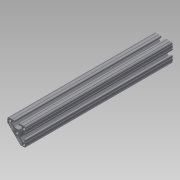
# Autodesk Inventor part: 1547
Saved by Autodesk Inventor 2013 (Build 170138000, 138)
## iProperties
Company: 80/20 Inc.
Created: 2014-04-23
Part Number: 1547
Material: Generic
Document SubType Name: Modeling
Density: 1 g/cm^3
Vendor: 80/20 Inc.
Engineer: Ross Bowman
Designer: Ross Bowman
Catalog Web Link: 8020.net
Material: 6105-T5 Aluminum
Author: Ross Bowman
Keywords: 80/20 , 8020 , T-Slot , Extrusion
Autodesk Inventor part; units mm, degrees
ref_plane "YZ Plane" through (0, 0, 0) normal (1, 0, 0) x (0, 1, 0)
ref_plane "XZ Plane" through (0, 0, 0) normal (0, 1, 0) x (-1, 0, 0)
ref_plane "XY Plane" through (0, 0, 0) normal (0, 0, 1) x (1, 0, 0)
sketch "Sketch1" plane through (0, 0, 0) normal (0, 0, 1) x (1, 0, 0)
  circle A0 centre (0, 0) radius 3.3274
  arc A1 (12.2428, 17.272) -> (11.8618, 16.891) centre (12.2428, 16.891) ccw
  line L0 (14.478, 17.272) -> (12.2428, 17.272)
  arc A2 (17.272, 14.478) -> (14.478, 17.272) centre (14.478, 14.478) ccw
  line L1 (17.272, 12.2682) -> (17.272, 14.478)
  arc A3 (16.891, 11.8872) -> (17.272, 12.2682) centre (16.891, 12.2682) ccw
  line L2 (12.2428, 11.8872) -> (16.891, 11.8872)
  arc A4 (11.8618, 12.2682) -> (12.2428, 11.8872) centre (12.2428, 12.2682) ccw
  line L3 (11.8618, 16.891) -> (11.8618, 12.2682)
  arc A5 (-12.2428, 11.8872) -> (-11.8618, 12.2682) centre (-12.2428, 12.2682) ccw
  line L4 (-16.8656, 11.8872) -> (-12.2428, 11.8872)
  arc A6 (-17.2466, 12.2682) -> (-16.8656, 11.8872) centre (-16.8656, 12.2682) ccw
  line L5 (-17.2466, 14.478) -> (-17.2466, 12.2682)
  arc A7 (-14.4526, 17.272) -> (-17.2466, 14.478) centre (-14.4526, 14.478) ccw
  line L6 (-12.2428, 17.272) -> (-14.4526, 17.272)
  arc A8 (-11.8618, 16.891) -> (-12.2428, 17.272) centre (-12.2428, 16.891) ccw
  line L7 (-11.8618, 12.2682) -> (-11.8618, 16.891)
  arc A9 (14.478, -17.272) -> (17.272, -14.478) centre (14.478, -14.478) ccw
  line L8 (12.2428, -17.272) -> (14.478, -17.272)
  arc A10 (11.8618, -16.891) -> (12.2428, -17.272) centre (12.2428, -16.891) ccw
  line L9 (11.8618, -12.2682) -> (11.8618, -16.891)
  arc A11 (12.2428, -11.8872) -> (11.8618, -12.2682) centre (12.2428, -12.2682) ccw
  line L10 (16.891, -11.8872) -> (12.2428, -11.8872)
  arc A12 (17.272, -12.2682) -> (16.891, -11.8872) centre (16.891, -12.2682) ccw
  line L11 (17.272, -14.478) -> (17.272, -12.2682)
  arc A13 (10.287, -12.9937) -> (9.915, -12.0957) centre (9.017, -12.9937) ccw
  line L12 (10.287, -16.6116) -> (10.287, -12.9937)
  arc A14 (9.525, -17.3736) -> (10.287, -16.6116) centre (9.525, -16.6116) ccw
  line L13 (8.7106, -17.3736) -> (9.525, -17.3736)
  arc A15 (8.1718, -17.1504) -> (8.7106, -17.3736) centre (8.7106, -16.6116) ccw
  line L14 (-0.94, -8.0387) -> (8.1718, -17.1504)
  arc A16 (-0.4088, -6.7564) -> (-0.94, -8.0387) centre (-0.4088, -7.5076) ccw
  line L15 (2.6083, -6.7564) -> (-0.4088, -6.7564)
  arc A17 (5.9669, -8.1476) -> (2.6083, -6.7564) centre (2.6083, -11.5062) ccw
  line L16 (9.915, -12.0957) -> (5.9669, -8.1476)
  arc A18 (-8.0318, -0.9468) -> (-6.731, -0.408) centre (-7.493, -0.408) ccw
  line L17 (-17.1758, 8.1972) -> (-8.0318, -0.9468)
  arc A19 (-17.399, 8.736) -> (-17.1758, 8.1972) centre (-16.637, 8.736) ccw
  line L18 (-17.399, 9.5504) -> (-17.399, 8.736)
  arc A20 (-16.637, 10.3124) -> (-17.399, 9.5504) centre (-16.637, 9.5504) ccw
  line L19 (-12.9683, 10.3124) -> (-16.637, 10.3124)
  arc A21 (-12.0703, 9.9404) -> (-12.9683, 10.3124) centre (-12.9683, 9.0424) ccw
  line L20 (-8.1222, 5.9923) -> (-12.0703, 9.9404)
  arc A22 (-6.731, 2.6337) -> (-8.1222, 5.9923) centre (-11.4808, 2.6337) ccw
  line L21 (-6.731, -0.408) -> (-6.731, 2.6337)
  arc A23 (19.05, 15.7774) -> (19.05, 14.3289) centre (19.05, 15.0532) ccw
  line L22 (19.05, 15.7774) -> (19.05, 15.875)
  arc A24 (19.05, 15.875) -> (15.7653, 19.05) centre (15.875, 15.8769) ccw
  arc A25 (14.0827, 19.05) -> (15.7653, 19.05) centre (14.924, 19.05) ccw
  line L23 (14.0827, 19.05) -> (9.1655, 19.05)
  arc A26 (7.8261, 19.05) -> (9.1655, 19.05) centre (8.4958, 19.05) ccw
  line L24 (7.8261, 19.05) -> (5.6388, 19.05)
  arc A27 (5.6388, 19.05) -> (4.064, 17.4752) centre (5.6388, 17.4752) ccw
  line L25 (4.064, 17.4752) -> (4.064, 16.5608)
  arc A28 (4.064, 16.5608) -> (5.6388, 14.986) centre (5.6388, 16.5608) ccw
  line L26 (5.6388, 14.986) -> (6.5869, 14.986)
  arc A29 (6.5869, 14.986) -> (6.9518, 15.4766) centre (6.5869, 15.367) ccw
  arc A30 (7.3166, 15.9672) -> (6.9518, 15.4766) centre (7.3166, 15.5862) ccw
  line L27 (7.3166, 15.9672) -> (9.017, 15.9672)
  arc A31 (10.287, 14.6972) -> (9.017, 15.9672) centre (9.017, 14.6972) ccw
  line L28 (10.287, 14.6972) -> (10.287, 12.9937)
  arc A32 (9.915, 12.0957) -> (10.287, 12.9937) centre (9.017, 12.9937) ccw
  line L29 (9.915, 12.0957) -> (5.9669, 8.1476)
  arc A33 (2.6083, 6.7564) -> (5.9669, 8.1476) centre (2.6083, 11.5062) ccw
  line L30 (2.6083, 6.7564) -> (-2.6083, 6.7564)
  arc A34 (-5.9669, 8.1476) -> (-2.6083, 6.7564) centre (-2.6083, 11.5062) ccw
  line L31 (-5.9669, 8.1476) -> (-9.915, 12.0957)
  arc A35 (-10.287, 12.9937) -> (-9.915, 12.0957) centre (-9.017, 12.9937) ccw
  line L32 (-10.287, 12.9937) -> (-10.287, 14.6972)
  arc A36 (-9.017, 15.9672) -> (-10.287, 14.6972) centre (-9.017, 14.6972) ccw
  line L33 (-9.017, 15.9672) -> (-7.4834, 15.9672)
  arc A37 (-7.1185, 15.4766) -> (-7.4834, 15.9672) centre (-7.4834, 15.5862) ccw
  arc A38 (-7.1185, 15.4766) -> (-6.7536, 14.986) centre (-6.7536, 15.367) ccw
  line L34 (-6.7536, 14.986) -> (-5.6388, 14.986)
  arc A39 (-5.6388, 14.986) -> (-4.064, 16.5608) centre (-5.6388, 16.5608) ccw
  line L35 (-4.064, 16.5608) -> (-4.064, 17.4752)
  arc A40 (-4.064, 17.4752) -> (-5.6388, 19.05) centre (-5.6388, 17.4752) ccw
  line L36 (-5.6388, 19.05) -> (-8.2517, 19.05)
  arc A41 (-9.5563, 19.05) -> (-8.2517, 19.05) centre (-8.904, 19.05) ccw
  line L37 (-9.5563, 19.05) -> (-14.6013, 19.05)
  arc A42 (-15.9068, 19.05) -> (-14.6013, 19.05) centre (-15.254, 19.05) ccw
  arc A43 (-15.9068, 19.05) -> (-19.05, 15.9297) centre (-15.8755, 15.8752) ccw
  arc A44 (-19.05, 14.5315) -> (-19.05, 15.9297) centre (-19.05, 15.2306) ccw
  line L38 (-19.05, 14.5315) -> (-19.05, 8.3493)
  arc A45 (-19.05, 8.3493) -> (-18.8268, 7.8105) centre (-18.288, 8.3493) ccw
  line L39 (-18.8268, 7.8105) -> (-16.787, 5.7706)
  arc A46 (-15.7093, 4.693) -> (-16.787, 5.7706) centre (-16.2482, 5.2318) ccw
  line L40 (-15.7093, 4.693) -> (-12.2968, 1.2805)
  arc A47 (-11.2192, 0.2029) -> (-12.2968, 1.2805) centre (-11.758, 0.7417) ccw
  line L41 (-11.2192, 0.2029) -> (0.0599, -11.0762)
  arc A48 (1.1375, -12.1539) -> (0.0599, -11.0762) centre (0.5987, -11.6151) ccw
  line L42 (1.1375, -12.1539) -> (4.55, -15.5664)
  arc A49 (5.6277, -16.644) -> (4.55, -15.5664) centre (5.0888, -16.1052) ccw
  line L43 (5.6277, -16.644) -> (7.8105, -18.8268)
  arc A50 (7.8105, -18.8268) -> (8.3493, -19.05) centre (8.3493, -18.288) ccw
  line L44 (8.3493, -19.05) -> (14.6389, -19.05)
  arc A51 (15.7557, -19.05) -> (14.6389, -19.05) centre (15.1973, -19.05) ccw
  line L45 (15.7557, -19.05) -> (15.7811, -19.05)
  arc A52 (15.7811, -19.05) -> (19.05, -15.7851) centre (15.8763, -15.8764) ccw
  line L46 (19.05, -15.7851) -> (19.05, -15.7501)
  arc A53 (19.05, -14.5319) -> (19.05, -15.7501) centre (19.05, -15.141) ccw
  line L47 (19.05, -14.5319) -> (19.05, -9.5039)
  arc A54 (19.05, -7.9799) -> (19.05, -9.5039) centre (19.05, -8.7419) ccw
  line L48 (19.05, -7.9799) -> (19.05, -5.6981)
  arc A55 (19.05, -5.6981) -> (17.4752, -4.1233) centre (17.4752, -5.6981) ccw
  line L49 (17.4752, -4.1233) -> (16.5608, -4.1233)
  arc A56 (16.5608, -4.1233) -> (14.986, -5.6981) centre (16.5608, -5.6981) ccw
  line L50 (14.986, -5.6981) -> (14.986, -6.5363)
  arc A57 (14.986, -6.5363) -> (15.4065, -6.9152) centre (15.367, -6.5363) ccw
  arc A58 (15.8272, -7.2945) -> (15.4065, -6.9152) centre (15.4459, -7.2945) ccw
  line L51 (15.8272, -7.2945) -> (15.8272, -9.0424)
  arc A59 (14.5572, -10.3124) -> (15.8272, -9.0424) centre (14.5572, -9.0424) ccw
  line L52 (14.5572, -10.3124) -> (12.9683, -10.3124)
  arc A60 (12.0703, -9.9404) -> (12.9683, -10.3124) centre (12.9683, -9.0424) ccw
  line L53 (12.0703, -9.9404) -> (8.1222, -5.9923)
  arc A61 (6.731, -2.6337) -> (8.1222, -5.9923) centre (11.4808, -2.6337) ccw
  line L54 (6.731, -2.6337) -> (6.731, 2.6337)
  arc A62 (8.1222, 5.9923) -> (6.731, 2.6337) centre (11.4808, 2.6337) ccw
  line L55 (8.1222, 5.9923) -> (12.0703, 9.9404)
  arc A63 (12.9683, 10.3124) -> (12.0703, 9.9404) centre (12.9683, 9.0424) ccw
  line L56 (12.9683, 10.3124) -> (14.5572, 10.3124)
  arc A64 (15.8272, 9.0424) -> (14.5572, 10.3124) centre (14.5572, 9.0424) ccw
  line L57 (15.8272, 9.0424) -> (15.8272, 7.2945)
  arc A65 (15.4065, 6.9152) -> (15.8272, 7.2945) centre (15.4459, 7.2945) ccw
  arc A66 (15.4065, 6.9152) -> (14.986, 6.5363) centre (15.367, 6.5363) ccw
  line L58 (14.986, 6.5363) -> (14.986, 5.6981)
  arc A67 (14.986, 5.6981) -> (16.5608, 4.1233) centre (16.5608, 5.6981) ccw
  line L59 (16.5608, 4.1233) -> (17.4752, 4.1233)
  arc A68 (17.4752, 4.1233) -> (19.05, 5.6981) centre (17.4752, 5.6981) ccw
  line L60 (19.05, 5.6981) -> (19.05, 7.982)
  arc A69 (19.05, 9.5018) -> (19.05, 7.982) centre (19.05, 8.7419) ccw
  line L61 (19.05, 9.5018) -> (19.05, 14.3289)
  constraints: 138 point on circle, 124 end point, 70 centre point
extrude "Extrusion1" add sketch "Sketch1" against normal blind 304.8
body "Solid1"
